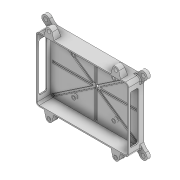
# Autodesk Inventor part: scatola - corpo sotto
Saved by Autodesk Inventor 2022 (Build 260153000, 153)
## iProperties
Created: 2025-07-13
Part Number: scatola - corpo sotto
Material: Generic
Document SubType Name: Modeling
Designer: 1234
Density: 1 g/cm^3
Appearance: Default
Author: 1234
Autodesk Inventor part; units mm, degrees
ref_plane "YZ Plane" through (0, 0, 0) normal (1, 0, 0) x (0, 1, 0)
ref_plane "XZ Plane" through (0, 0, 0) normal (0, 1, 0) x (-1, 0, 0)
ref_plane "XY Plane" through (0, 0, 0) normal (0, 0, 1) x (1, 0, 0)
sketch "Sketch1" plane through (0, 0, 0) normal (0, 0, 1) x (1, 0, 0)
  arc A0 (-4, 0) -> (0, -4) centre (0, 0) ccw
  circle A1 centre (0, 0) radius 1.6 construction
  circle A2 centre (0, 72) radius 1.6 construction
  arc A3 (0, 76) -> (-4, 72) centre (0, 72) ccw
  arc A4 (107, -4) -> (111, 0) centre (107, 0) ccw
  circle A5 centre (107, 0) radius 1.6 construction
  arc A6 (111, 72) -> (107, 76) centre (107, 72) ccw
  circle A7 centre (107, 72) radius 1.6 construction
  line L0 (111, 72) -> (111, 0)
  line L1 (107, 76) -> (0, 76)
  line L2 (-4, 72) -> (-4, 0)
  line L3 (0, -4) -> (107, -4)
  line L4 (-4, 36) -> (-11, 36) construction
  circle A8 centre (-11, 36) radius 2.3
  arc A9 (-11, 40) -> (-11, 32) centre (-11, 36) ccw
  line L5 (-11, 32) -> (-4, 32)
  line L6 (-11, 40) -> (-4, 40)
  line L7 (8, -4) -> (8, -11)
  arc A10 (8, -11) -> (16, -11) centre (12, -11) ccw
  line L8 (16, -11) -> (16, -4)
  circle A11 centre (12, -11) radius 2.3
  line L9 (18, -4) -> (15.8657, -12.0278)
  line L10 (6, -4) -> (8.1343, -12.0278)
  line L11 (-12.0278, 32.1343) -> (-4, 30)
  line L12 (-12.0278, 39.8657) -> (-4, 42)
  line L13 (18, 76) -> (15.8657, 84.0278)
  line L14 (16, 83) -> (16, 76)
  arc A12 (16, 83) -> (8, 83) centre (12, 83) ccw
  circle A13 centre (12, 83) radius 2.3
  line L15 (8, 76) -> (8, 83) construction
  line L16 (8, 83) -> (8, 76)
  line L17 (6, 76) -> (8.1343, 84.0278)
  line L18 (0, 72) -> (107, 72) construction
  line L19 (107, 0) -> (107, 72) construction
  line L20 (0, 72) -> (0, 0) construction
  line L21 (0, 0) -> (107, 0) construction
  arc A14 (0, 74.5) -> (-2.5, 72) centre (0, 72) ccw
  line L22 (-2.5, 72) -> (-2.5, 0)
  arc A15 (-2.5, 0) -> (0, -2.5) centre (0, 0) ccw
  line L23 (0, -2.5) -> (107, -2.5)
  arc A16 (107, -2.5) -> (109.5, 0) centre (107, 0) ccw
  line L24 (109.5, 0) -> (109.5, 72)
  arc A17 (109.5, 72) -> (107, 74.5) centre (107, 72) ccw
  line L25 (107, 74.5) -> (0, 74.5)
  circle A18 centre (-7.0711, 79.0711) radius 2.5
  circle A19 centre (-7.0711, 79.0711) radius 5
  line L26 (0, 72) -> (-15.7171, 87.7171) construction
  arc A20 (-2.7655, 81.6131) -> (4, 76) centre (8.4291, 88.2222) ccw
  arc A21 (-4, 68) -> (-9.6131, 74.7655) centre (-16.2222, 63.5709) ccw
  dimension "d38" = 3.2
  dimension "d39" = 3.2
  dimension "d41" = 3.2
  dimension "d68" = 7
  dimension "d69" = 4.6
  dimension "d70" = 8
  dimension "d71" = 8
  dimension "d72" = 7
  dimension "d73" = 4.6
  dimension "d74" = 2
  dimension "d75" = 2
  dimension "d76" = 2
  dimension "d77" = 2
  dimension "d78" = 4
  dimension "d79" = 4
  dimension "d80" = 4
  dimension "d81" = 4
  dimension "d83" = 107
  dimension "d84" = 72
  dimension "d87" = 8
  dimension "d93" = 1.5
  dimension "d194" = 5
  dimension "d195" = 10
  dimension "d196" = 10
  dimension "d197" = 135
  dimension "d199" = 13
  dimension "d200" = 4
  dimension "d201" = 4
  dimension "d202" = 13
  constraints: 59 end point, 34 point on circle, 22 centre point, 15 tangent, 13 point on line, 10 symmetric about line, 9 coincident, 5 horizontal, 4 vertical, 2 perpendicular, 1 equal radius, 1 midpoint, 10 other
  measures "d38" diameter of A5
  measures "d39" diameter of A7
  measures "d41" diameter of A1
  measures "d68" distance of L4.start L4.end
  measures "d69" diameter of A8
  measures "d70" diameter of A9
  measures "d71" diameter of A10
  measures "d72" distance from line of A10.centre L3
  measures "d73" diameter of A11
  measures "d74" distance of L9.start L8.end
  measures "d75" distance from line of L7 L10.start
  measures "d76" distance of L11.end L5.end
  measures "d77" distance from line of L6 L12.end
  measures "d78" radius of A6
  measures "d79" radius of A4
  measures "d80" radius of A0
  measures "d81" radius of A3
  measures "d83" distance between parallel lines of L19 L20
  measures "d84" distance between parallel lines of L18 L21
  measures "d87" distance between parallel lines of L20 L7
  measures "d93" distance between parallel lines of L1 L25
  measures "d194" diameter of A18
  measures "d195" diameter of A19
  measures "d196" distance of L20.start A18.centre
  measures "d197" angle of L20 L26
  measures "d199" radius of A20
  measures "d200" distance from line of L20 A20.end
  measures "d201" distance from line of A21.start L18
  measures "d202" radius of A21
extrude "Extrusion1" add sketch "Sketch1" along normal blind 2 contours L2 A3 L1 A6 L0 A4 L3 A0 | L25 A17 L24 A16 L23 A15 L22 A14
extrude "Extrusion3" add sketch "Sketch1" along normal blind 19 contours L2 A3 L1 A6 L0 A4 L3 A0
ref_plane "Work Plane7" through (0, 0, 12) normal (0, 0, 1) x (1, 0, 0)
extrude "Extrusion2" add sketch "Sketch1" along normal up to surface (7 mm away) from surface at 12 contours L3 L7 A10 L10 | L3 L8 A10 L7 | L3 L9 A10 L8 | L17 A12 L16 L1 | L1 L14 A12 L13 | L16 A12 L14 L1
ref_plane "Work Plane1" through (53.5, 0, 0) normal (1, 0, 0) x (0, 0, -1)
chamfer "Chamfer12" distance 2 distance2 9 1 edges at (12, 76, 12) measured on face at (12, 76, 11.5)
chamfer "Chamfer13" distance 2 distance2 9 1 edges at (12, -4, 12) measured on face at (12, -4, 11.5)
mirror "Mirror1" about plane through (53.5, 0, 0) normal (1, 0, 0) of "Extrusion2", "Chamfer12", "Chamfer13"
sketch "Sketch2" plane through (0, 0, 2) normal (0, 0, 1) x (1, 0, 0)
  arc A0 (0, 74.5) -> (-2.5, 72) centre (0, 72) ccw projected
  arc A1 (107, -2.5) -> (109.5, 0) centre (107, 0) ccw projected
  line L0 (0, 72) -> (107, 0) construction
  arc A2 (109.5, 72) -> (107, 74.5) centre (107, 72) ccw projected
  line L1 (0, 0) -> (107, 72) construction
  circle A3 centre (53.5, 36) radius 1.5
  line L2 (53.5, 36) -> (53.5, 72) construction
  line L3 (53.5, 36) -> (53.5, 0) construction
  line L4 (53.5, 36) -> (107, 36) construction
  line L5 (53.5, 36) -> (0, 36) construction
  line L6 (-0.5583, 71.1703) -> (106.4417, -0.8297)
  line L7 (0.5583, 72.8297) -> (107.5583, 0.8297)
  line L8 (52.5, 36) -> (52.5, 72)
  line L9 (54.5, 36) -> (54.5, 72)
  line L10 (-0.5583, 0.8297) -> (106.4417, 72.8297)
  line L11 (0.5583, -0.8297) -> (107.5583, 71.1703)
  line L12 (54.5, 36) -> (54.5, 0)
  line L13 (52.5, 36) -> (52.5, 0)
  line L14 (-0.5583, 0.8297) -> (0.5583, -0.8297)
  line L15 (-0.5583, 71.1703) -> (0.5583, 72.8297)
  line L16 (52.5, 72) -> (54.5, 72)
  line L17 (106.4417, 72.8297) -> (107.5583, 71.1703)
  line L18 (53.1088, 37) -> (107, 37)
  line L19 (53.5, 35) -> (107, 35)
  line L20 (53.5, 35) -> (0, 35)
  line L21 (53.3915, 37) -> (0, 37)
  line L22 (0, 37) -> (0, 35)
  line L23 (107, 35) -> (107, 37)
  line L24 (106.4417, -0.8297) -> (107.5583, 0.8297)
  line L25 (52.5, 0) -> (54.5, 0)
  arc A4 (-2.5, 0) -> (0, -2.5) centre (0, 0) ccw projected
  circle A5 centre (0, 0) radius 2.5 construction
  line L26 (107, 0) -> (107, 72) construction
  line L27 (0, 72) -> (0, 0) construction
  line L28 (107, 72) -> (0, 72) construction
  line L29 (0, 0) -> (107, 0) construction
  point P0 (50.2227, 35)
  point P1 (52.5, 34.1218)
  point P2 (54.5, 34.1218)
  point P3 (56.7773, 35)
  point P4 (56.7773, 37)
  point P5 (75.8056, 46.2872)
  point P6 (54.5, 37.8782)
  point P7 (52.5, 37.8782)
  point P8 (15.3318, 56.2198)
  point P9 (50.2227, 37)
  point P10 (53.5, 34.7947)
  point P11 (53.8693, 34.5462)
  point P12 (53.1307, 34.5462)
  point P13 (53.1949, 37)
  point P14 (53.8051, 37)
  point P15 (54.5, 36.5324)
  point P16 (54.5, 35.4676)
  point P17 (53.8051, 35)
  point P18 (53.1949, 35)
  point P19 (52.5, 35.4676)
  point P20 (52.5, 36.5324)
  dimension "d98" = 3
  dimension "d101" = 1
  dimension "d102" = 1
  dimension "d103" = 1
  dimension "d104" = 1
  dimension "d105" = 1
  dimension "d106" = 1
  dimension "d107" = 1
  dimension "d108" = 1
  dimension "d109" = 1
  dimension "d110" = 1
  dimension "d111" = 1
  dimension "d112" = 1
  constraints: 60 end point, 12 parallel, 10 midpoint, 6 vertical, 5 perpendicular, 4 collinear, 4 horizontal, 1 centre point, 1 coincident, 1 horizontal alignment, 2 other
  measures "d98" diameter of A3
  measures "d101" distance between parallel lines of L0 L6
  measures "d102" distance between parallel lines of L0 L7
  measures "d103" distance between parallel lines of L2 L8
  measures "d104" distance between parallel lines of L2 L9
  measures "d105" distance between parallel lines of L1 L10
  measures "d106" distance between parallel lines of L1 L11
  measures "d107" distance between parallel lines of L3 L12
  measures "d108" distance between parallel lines of L3 L13
  measures "d109" distance between parallel lines of L4 L18
  measures "d110" distance between parallel lines of L4 L19
  measures "d111" distance between parallel lines of L5 L20
  measures "d112" distance between parallel lines of L5 L21
extrude "Extrusion4" cut sketch "Sketch2" against normal through all contours A3 L11 L12 L9 L7 | L7 L9 L18 A3 | A3 L19 L12 L11 | L18 L9 A3 | L9 L12 L11 L19 L20 L6 L13 L8 L10 L18 L7 | L7 L18 L9 | A3 L12 L19 | L12 L19 L11 | L9 L18 L7 L10 A3 | L18 L10 L7 | A3 L6 L11 L19 L12 | L11 L6 L20 L19 | L10 L7 A3 | L10 L18 L21 L8 A3 L7 | A3 L11 L6 | L11 A3 L13 L20 L6 | L10 L8 L21 L18 | L20 L13 L6 | L8 L21 A3 | L10 A3 L21 L8 | L8 L13 L6 A3 L10 | A3 L20 L13 | L13 L20 A3 L6
extrude "Extrusion5" cut sketch "Sketch2" against normal blind 1 contours A3 L7 L11 | A3 L18 L11 L7 | L11 L7 L19 A3 | A3 L9 L10 L17 L11 L18 | L11 L18 L23 L19 L7 | L19 L7 L24 L6 L12 A3 | A3 L10 L9 | L12 L6 A3 | A3 L7 L8 L16 L9 L10 | L6 L12 L25 L13 L11 A3 | A3 L11 L6 | A3 L8 L7 | L11 L13 A3 | A3 L21 L6 L15 L7 L8 | L13 L11 L14 L10 L20 A3 | A3 L10 L6 L21 | A3 L6 L10 | L20 L10 L6 A3 | L6 L10 L20 L22 L21
sketch "Sketch3" plane through (111, 0, 0) normal (1, 0, 0) x (0, 0, -1)
  line L0 (-17, 6) -> (5.8153, 6) construction
  line L1 (5.8153, 66) -> (-17, 66) construction
  line L2 (0, -4) -> (-19, -4) projected
  line L3 (0, 76) -> (-19, 76) projected
  line L4 (-19, 6) -> (-19, 66)
  line L5 (-7, 66) -> (-7, 6)
  line L6 (-19, 6) -> (-7, 6)
  line L7 (-7, 66) -> (-19, 66)
  line L8 (-19, 0) -> (-19, 72) projected
  line L9 (-17, 6) -> (-17, 66)
  point P0 (0, 0)
  dimension "d115" = 10
  dimension "d116" = 10
  dimension "d117" = 12
  dimension "d118" = 0
  dimension "d215" = 2
  constraints: 14 end point, 6 point on line, 3 perpendicular, 2 horizontal, 1 vertical, 1 other
  measures "d115" distance between parallel lines of L2 L0
  measures "d116" distance between parallel lines of L3 L1
  measures "d117" distance between parallel lines of L4 L5
  measures "d118" horizontal extent of L4
  measures "d215" distance between parallel lines of L4 L9
extrude "Extrusion6" cut sketch "Sketch3" against normal through all contours L9 L7 L5 L6
sketch "Sketch4" plane through (0, 0, 2) normal (0, 0, 1) x (1, 0, 0)
  circle A0 centre (28.5, 59) radius 2.5
  circle A1 centre (78.5, 59) radius 2.5
  line L0 (-2.5, 0) -> (-2.5, 72) projected
  line L1 (0, 74.5) -> (107, 74.5) projected
  line L2 (109.5, 6) -> (109.5, 66) projected
  circle A2 centre (53.5, 36) radius 1.5 projected
  line L3 (53.5, 36) -> (107, 36) construction
  line L4 (107, 37) -> (107, 35) projected
  circle A3 centre (28.5, 59) radius 1.4
  circle A4 centre (78.5, 59) radius 1.4
  circle A5 centre (28.5, 13) radius 2.5
  circle A6 centre (78.5, 13) radius 2.5
  circle A7 centre (28.5, 13) radius 1.4
  circle A8 centre (78.5, 13) radius 1.4
  line L5 (27.1, 59) -> (82.8154, 59) construction
  line L6 (53.5, 36) -> (53.5, 69.5) construction
  point P0 (-2.5, 46)
  point P1 (-2.5, 52)
  point P2 (0, 54.5)
  point P3 (72, 54.5)
  dimension "d190" = 2.8
  dimension "d184" = 5
  dimension "d185" = 5
  dimension "d191" = 2.8
  dimension "d220" = 46
  dimension "d221" = 50
  dimension "d222" = 25
  constraints: 7 centre point, 6 end point, 4 coincident, 4 symmetric about line, 2 point on line, 1 horizontal, 1 horizontal alignment, 1 midpoint, 1 vertical, 7 other
  measures "d184" diameter of A1
  measures "d185" diameter of A0
  measures "d191" diameter of A4
  measures "d220" distance of A0.centre A5.centre
  measures "d221" distance of A1.centre A0.centre
  measures "d222" distance from line of L6 A0.centre
extrude "Extrusion7" add sketch "Sketch4" along normal blind 3 contours A0 | A1 | A5 | A6
fillet "Fillet1" radius 0.6 8 edges at (50.2227, 37, 1.5) (52.5, 37.8782, 1.5) (54.5, 37.8782, 1.5) (56.7773, 37, 1.5) (56.7773, 35, 1.5) (54.5, 34.1218, 1.5) (52.5, 34.1218, 1.5) (50.2227, 35, 1.5)
chamfer "Chamfer1" distance 0.6 angle 45 33 edges at (24.0165, 17.3659, 2) (48.8301, 34.5751, 2) (24.1281, 35, 2) (52.182, 33.5245, 2) (52.5, 16.4974, 2) (26.0617, 16.3315, 2) (82.8719, 35, 2) (58.1699, 34.5751, 2) (82.9835, 17.3659, 2) (80.9383, 16.3315, 2) (54.818, 33.5245, 2) (54.5, 16.4974, 2) (80.9383, 55.6685, 2) (54.818, 38.4755, 2) (54.5, 55.5026, 2) (82.9835, 54.6341, 2) (58.1699, 37.4249, 2) (82.8719, 37, 2) (52.5, 55.5026, 2) (52.182, 38.4755, 2) (26.0617, 55.6685, 2) (24.0165, 54.6341, 2) (48.8301, 37.4249, 2) (24.1281, 37, 2) (0, 0, 2) (0, 36, 2) (0, 72, 2) (53.5, 0, 2) (107, 0, 2) (107, 36, 2) (107, 72, 2) (53.5, 72, 2) (52, 36, 1)
fillet "Fillet2" radius 2 8 edges at (-3.25, 66, 7) (110.25, 66, 7) (110.25, 6, 7) (-3.25, 6, 7) (-3.25, 66, 17) (-3.25, 6, 17) (110.25, 6, 17) (110.25, 66, 17)
extrude "Extrusion9" cut sketch "Sketch4" against normal through all contours A3 | A4 | A7 | A8
extrude "Extrusion10" add sketch "Sketch1" along normal blind 4 contours A21 A19 A20 L1 A3 L2 | A19
mirror "Mirror3" about plane through (53.5, 0, 0) normal (1, 0, 0) of "Extrusion10"
ref_plane "Work Plane6" through (0, 36, 0) normal (0, -1, 0) x (1, 0, 0)
mirror "Mirror4" about plane through (0, 36, 0) normal (0, -1, 0) of "Extrusion10", "Mirror3"
chamfer "Chamfer11" distance 1 angle 45 12 edges at (-4, 70, 4) (-2.8284, 74.8284, 4) (2, 76, 4) (109.8284, 74.8284, 4) (105, 76, 4) (111, 70, 4) (109.8284, -2.8284, 4) (111, 2, 4) (105, -4, 4) (-2.8284, -2.8284, 4) (2, -4, 4) (-4, 2, 4)
equation "\"d39\" = d38"
equation "\"d41\" = d38"
equation "\"d74\" = d75"
equation "\"d76\" = d75"
equation "\"d77\" = d75"
body "Solid1"
